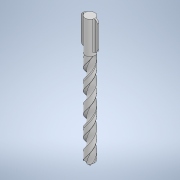
# Autodesk Inventor part: Część10
Saved by Autodesk Inventor 2021 (Build 250183000, 183)
## iProperties
Created: 2023-09-29
Part Number: Część10
Material: Ogólny
Document SubType Name: Modeling
Designer: Jakub
Density: 1 g/cm^3
Appearance: Domyślna
Author: Jakub
Autodesk Inventor part; units mm, degrees
ref_plane "YZ Plane" through (0, 0, 0) normal (1, 0, 0) x (0, 1, 0)
ref_plane "XZ Plane" through (0, 0, 0) normal (0, 1, 0) x (-1, 0, 0)
ref_plane "XY Plane" through (0, 0, 0) normal (0, 0, 1) x (1, 0, 0)
sketch "Szkic1" plane through (0, 0, 0) normal (0, 1, 0) x (-1, 0, 0)
  line L0 (0, 0) -> (0, -3)
  line L1 (0, -3) -> (3, -3)
  line L2 (3, -3) -> (3, 3)
  line L3 (3, 3) -> (-3, 3)
  line L4 (-3, 3) -> (-3, -3)
  line L5 (-3, -3) -> (0, -3)
  dimension "d0" = 3
  dimension "d1" = 3
  dimension "d2" = 6
  dimension "d3" = 6
  constraints: 12 end point, 5 perpendicular, 1 point on line, 1 vertical
  measures "d0" distance of L0.start L0.end
  measures "d1" distance of L0.end L1.end
  measures "d2" distance of L1.end L2.end
  measures "d3" distance of L2.end L3.end
extrude "Wyciągnięcie proste1" add sketch "Szkic1" along normal blind 20
sketch "Szkic3" plane through (-3, 0, -3) normal (-1, 0, 0) x (0, 0, 1)
  line L0 (3.5, 0) -> (2.5, 0) construction
  line L1 (2.5, 20) -> (2.5, 0) projected
  line L2 (2.5, 0) -> (2.5, 20)
  line L3 (2.5, 20) -> (3.5, 20) projected
  line L4 (2.5, 20) -> (3.5, 20)
  line L5 (3.5, 0) -> (3.5, 20) projected
  line L6 (3.5, 20) -> (3.5, 0)
  line L7 (3.5, 0) -> (2.5, 0)
  line L8 (2.5, 2) -> (3.5, 2)
  point P0 (3, 0)
  constraints: 10 end point, 3 perpendicular, 2 point on line, 1 collinear, 1 vertical
extrude "Wyciągnięcie proste3" add sketch "Szkic3" along normal blind 2 contours L3 L5 L8 L1
sketch "Szkic4" plane through (3, 0, 3) normal (1, 0, 0) x (0, 0, -1)
  line L0 (3.5, 20) -> (3.5, 2) projected
  line L1 (3.5, 20) -> (3.5, 2)
  line L2 (3.5, 2) -> (2.5, 2) projected
  line L3 (3.5, 2) -> (2.5, 2)
  line L4 (2.5, 2) -> (2.5, 20) projected
  line L5 (2.5, 2) -> (2.5, 20)
  line L6 (2.5, 20) -> (3.5, 20)
  line L7 (0, 20) -> (6, 20) projected
  point P0 (3, 0)
  constraints: 8 end point, 2 collinear, 2 perpendicular
extrude "Wyciągnięcie proste4" add sketch "Szkic4" along normal blind 2
fillet "Zaokrąglenie1" radius 3 1 edges at (3, 10, -3)
fillet "Zaokrąglenie2" radius 3 3 edges at (3, 10, 3) (-3, 10, -3) (-3, 10, 3)
fillet "Zaokrąglenie3" radius 2 4 edges at (-5, 2, 0) (5, 2, 0) (-5, 20, 0) (5, 20, 0)
fillet "Zaokrąglenie4" radius 1 4 edges at (2.9581, 11, 0.5) (2.958, 11, -0.5) (-2.9581, 11, -0.5) (-2.9581, 11, 0.5)
sketch "Szkic7" plane through (0, 0, 0) normal (0, -1, 0) x (1, 0, 0)
  point P0 (0, 0)
sketch "Szkic11" plane through (0, 0, 0) normal (0, -1, 0) x (1, 0, 0)
  line L0 (0, 0) -> (2.5, 0)
  line L1 (2.5, 0) -> (-2.5, 0)
  arc A0 (2.7811, 1.125) -> (-2.7811, 1.125) centre (0, 0) ccw projected
  line L2 (-0.5, 2.958) -> (-0.5, -3.042)
  line L3 (-0.5, 2.958) -> (5.5, 2.958) construction
  line L4 (0.5, 3) -> (0.5, -3)
  line L5 (0.5, 3) -> (6.5, 3) construction
  circle A1 centre (-2.5, 0) radius 1
  circle A2 centre (2.5, 0) radius 1
  line L6 (-1.5, 0) -> (-0.5, 2.958)
  line L7 (1.5, 0) -> (0.5, -2.958)
  arc A3 (-2.7811, -1.125) -> (2.7811, -1.125) centre (0, 0) ccw projected
  arc A4 (-2.7811, 1.125) -> (-3, 0) centre (0, 0) ccw projected
  arc A5 (-0.5, 2.958) -> (-2.85, 0.9367) centre (0, 0) ccw
  arc A6 (-3, 0) -> (-2.7811, -1.125) centre (0, 0) ccw projected
  arc A7 (-2.85, -0.9367) -> (-0.5, -2.958) centre (0, 0) ccw
  arc A8 (2.7811, -1.125) -> (3, 0) centre (0, 0) ccw projected
  arc A9 (0.5, -2.958) -> (2.85, -0.9367) centre (0, 0) ccw
  arc A10 (3, 0) -> (2.7811, 1.125) centre (0, 0) ccw projected
  arc A11 (2.85, 0.9367) -> (0.5, 2.958) centre (0, 0) ccw
  dimension "d53" = 2.5
  dimension "d54" = 5
  dimension "d59" = 6
  dimension "d60" = 90
  dimension "d61" = 6
  dimension "d62" = 90
  dimension "d63" = 2
  dimension "d64" = 2
  constraints: 21 point on circle, 16 end point, 7 point on line, 6 centre point, 6 coincident, 3 horizontal, 2 perpendicular
  measures "d53" distance of L0.start L0.end
  measures "d54" distance of L0.end L1.end
  measures "d59" distance of L2.start L2.end
  measures "d60" angle of L2 L3
  measures "d61" distance of L4.start L4.end
  measures "d62" angle of L4 L5
  measures "d63" diameter of A1
  measures "d64" diameter of A2
coil "Zwój1" sketch "Szkic11" operation add axis through (0, -10, 0) along (0, -1, 0) pitch 25 turns 2.4 hand right contours L1 L2 A0 L4 L0 | L0 L4 A3 L2 L1 | L4 A0 A10 A2 L0 | L0 L7 L4 | L2 A3 A6 A1 L1 | L1 L6 L2
sketch "Szkic18" plane through (0, 0, 0) normal (0, 0, 1) x (1, 0, 0)
  point P0 (0, 0)
sketch "Szkic19" plane through (0, 0, 0) normal (0, 0, 1) x (1, 0, 0)
  point P0 (0, 0)
sketch "Szkic20" plane through (0, 0, 0) normal (1, 0, 0) x (0, 1, 0)
  line L0 (-60, 0.7245) -> (-60, -2.687) projected
  line L1 (-60, -0.5) -> (-56.6434, -3.8566)
  line L2 (-60, -0.5) -> (-55.253, -0.5) construction
  line L3 (-56.6434, -3.8566) -> (-60, -3.8566)
  line L4 (-60, -3.8566) -> (-60, -0.5)
  line L5 (0, -5.3139) -> (0, 4.8873) projected
  line L6 (-76.0123, 0) -> (36.0036, 0) projected
  point P0 (0, 0)
  dimension "d85" = 45
  constraints: 8 end point, 1 collinear, 1 equal length, 1 horizontal, 1 perpendicular, 1 point on line
  measures "d85" angle of L1 L2
revolve "Obrót1" cut sketch "Szkic20" angle 360 about axis through (0, -10, 0) along (0, 1, 0)
